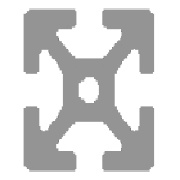
# Autodesk Inventor part: 40-4040
Saved by Autodesk Inventor 2016 (Build 200138000, 138)
## iProperties
IsCustomPart: 1
Created: 2015-07-26
Part Number: 40-4040
Material: Aluminum 6061
Document SubType Name: Modeling
Standard: 8020 Metric
Designer: myhome
Manufacturer: 8020
Standards Organization: 8020 Metric
Language: en-US
Size Designation: 40-4040
Categories: <MemberInstance><Categories><Category DisplayName="Structural Shapes" InternalName="089c4875-fa83-4c05-b084-43b9cc11f5ed" Mnemonic="GRDR"><CategoryParameter DisplayName="Mass per Length Unit" InternalName="0bb95a10-148f-4027-a459-38d7b056702a" Mnemonic="shpmass"/><CategoryParameter DisplayName="Section Area" InternalName="1ff91680-64b0-4202-b9a3-7fd3f94bba3b" Mnemonic="secarea"/><CategoryParameter DisplayName="Radius of Gyration (x)" InternalName="25778675-03e9-40c1-b6a8-4a9ed693320d" Mnemonic="gyrradx"/><CategoryParameter DisplayName="Torsional Rigidity Modulus" InternalName="26c1ec35-5026-4c63-ad0a-751cf684a536" Mnemonic="torrigmod"/><CategoryParameter DisplayName="Distance of the Center of Gravity X-X" InternalName="26c9bdb8-9c79-4b4f-a92e-8e197583c9c4" Mnemonic="grcendistX"/><CategoryParameter DisplayName="Legacy Member ID" InternalName="340afe4f-75d7-48d3-ab7d-943f3c3da468" Mnemonic="LegacyMemberID"/><CategoryParameter DisplayName="Base Length" InternalName="42e34263-8f20-4d0e-ad48-bf1385b87c24" Mnemonic="shplen"/><CategoryParameter DisplayName="Moment of Inertia (y)" InternalName="4b9f58ea-bced-460e-81ea-3d29ca5a49e3" Mnemonic="inermomy"/><CategoryParameter DisplayName="Moment of Inertia (x)" InternalName="4cd780bc-73d7-43ac-917a-579e5cbd684d" Mnemonic="inermomx"/><CategoryParameter DisplayName="Custom Base Point" InternalName="4f1d1b73-316d-484b-a3df-9cbabb16eb77" Mnemonic="shpBasePoint"/><CategoryParameter DisplayName="Shape Height" InternalName="50274e7d-5ac0-4796-92cb-c59e54983c67" Mnemonic="shpheig"/><CategoryParameter DisplayName="Section Module (y)" InternalName="59eaa5e9-d227-48dc-b6c1-6920f96e0f95" Mnemonic="secmody"/><CategoryParameter DisplayName="Section Designation" InternalName="5a64d034-428d-49c8-ba32-7619764de20f" Mnemonic="shpdes"/><CategoryParameter DisplayName="Section Module (x)" InternalName="72cfad18-cf51-4ed4-aaa7-c6b224f8419f" Mnemonic="secmodx"/><CategoryParameter DisplayName="Torsional Section Modulus" InternalName="7c55a8dc-8844-49f9-a867-cc677b30ec9a" Mnemonic="torsecmod"/><CategoryParameter DisplayName="Shape Width" InternalName="7c717d54-a18f-4666-b4d4-573cce22c62c" Mnemonic="shpwdth"/><CategoryParameter DisplayName="Second Shape Thickness" InternalName="9251a8e1-85fd-4e47-af99-afdb762317d9" Mnemonic="shpthick2"/><CategoryParameter DisplayName="FG Authored" InternalName="9c666724-f362-4ea7-ac62-f6a007de5c69" Mnemonic="shpFGAuto"/><CategoryParameter DisplayName="Distance of the Center of Gravity Y-Y" InternalName="bcc4fb17-7af4-436a-8f8c-d0aa3b0248c5" Mnemonic="grcendistY"/><CategoryParameter DisplayName="Radius of Gyration (y)" InternalName="bfa18ebe-1636-4dbe-8d42-b263e0b73184" Mnemonic="gyrrady"/><CategoryParameter DisplayName="Shape Thickness" InternalName="d109cf76-8eb4-42fc-9800-4409734adc67" Mnemonic="shpthick"/><CategoryParameter DisplayName="Coefficient of Shear Displacement" InternalName="de4c90c6-aaa8-468f-a335-6737b311b5d3" Mnemonic="shdispc"/><Category DisplayName="Other" InternalName="f02205ff-2390-476f-921c-0b3185f88e84" Mnemonic="OTHSHP"><CategoryParameter DisplayName="Moment of Inertia (y)" InternalName="044c654e-f649-48ac-84cc-650a29ae31ca" Mnemonic="inermomy"/><CategoryParameter DisplayName="Shape Thickness" InternalName="12b1a788-9233-48fd-a933-2df8ff42b15f" Mnemonic="shpthick"/><CategoryParameter DisplayName="Mass per Length Unit" InternalName="2fd289d6-9394-4d2d-97e6-6659d7d4551d" Mnemonic="shpmass"/><CategoryParameter DisplayName="Radius of Gyration (y)" InternalName="743e1dfe-1bba-408b-b985-cf752b207386" Mnemonic="gyrrady"/><CategoryParameter DisplayName="Section Module (y)" InternalName="88b8bff9-a616-4028-93d5-ed4f79680d13" Mnemonic="secmody"/><CategoryParameter DisplayName="Section Area" InternalName="c46ecdf8-b6eb-4db9-8b25-30258930c1e3" Mnemonic="secarea"/><CategoryParameter DisplayName="Section Module (x)" InternalName="cac70804-9d39-43bb-be17-56ea1f39a6c2" Mnemonic="secmodx"/><CategoryParameter DisplayName="Moment of Inertia (x)" InternalName="ec6737bc-264f-43ed-b0bd-f6d410c2718d" Mnemonic="inermomx"/><CategoryParameter DisplayName="Radius of Gyration (x)" InternalName="ee72c61e-565e-4fd6-b448-66e1e1abcb7e" Mnemonic="gyrradx"/><Category DisplayName="8020" InternalName="79851eee-1260-43d5-80eb-d25638456875" Mnemonic="8020"/></Category></Category><Category DisplayName="DataType" InternalName="23b78d0f-2648-40c6-8793-ca6db495c9e8" Mnemonic="DATATYPE"><CategoryParameter DisplayName="DisplayName" InternalName="05415f3d-3907-474b-a020-eb9d644f4cf3" Mnemonic="DISPLAYNAME"/><CategoryParameter DisplayName="Standard" InternalName="0c0a119c-1e12-4c84-803f-101930972f5e" Mnemonic="STANDARD"/><CategoryParameter DisplayName="Description" InternalName="13903e3d-64b1-4950-80da-f627842ea37f" Mnemonic="DESCRIPTION"/><CategoryParameter DisplayName="Designation" InternalName="2675968c-4ce5-49e0-a4f5-552d29089031" Mnemonic="DESIGNATION"/><CategoryParameter DisplayName="Default Row" InternalName="2af9ec52-faaa-4026-b378-f9fa4afca842" Mnemonic="DEFAULTROW"/><CategoryParameter DisplayName="Folder Name" InternalName="3f06958e-8713-4116-9be7-ed6184ecc97b" Mnemonic="FOLDERNAME"/><CategoryParameter DisplayName="Revision Guid" InternalName="45a75005-10b1-4dfc-8d6d-dfe629f0b93c" Mnemonic="REVISIONGUID"/><CategoryParameter DisplayName="FileName" InternalName="8b46a4cc-9585-4fed-90c3-899f57e09a73" Mnemonic="FILENAME"/><CategoryParameter DisplayName="StdsOrg" InternalName="8f5914e1-4693-403f-8ab5-d37768198c9d" Mnemonic="STDSORG"/><CategoryParameter DisplayName="Family Version" InternalName="914462f6-6e19-4b14-ba84-155b9680b1d0" Mnemonic="FAMILYREVISION"/><CategoryParameter DisplayName="Standard Revision" InternalName="91d5a463-65c2-4fde-b823-3b7fea5e8e17" Mnemonic="STANDARDREVISION"/><CategoryParameter DisplayName="Member Revision" InternalName="a65d44b9-392f-4f4f-857b-e4b3d54996fe" Mnemonic="MEMBERREVISION"/><CategoryParameter DisplayName="ClipFormat" InternalName="bc51e27b-3422-4e78-93ef-cec197ddf230" Mnemonic="CLIPFORMAT"/><CategoryParameter DisplayName="Manufacturer" InternalName="cd6c7a72-a28a-4e50-99a9-2c7f4e13e5ad" Mnemonic="MANUFACTURER"/><CategoryParameter DisplayName="InternalName" InternalName="cf1d0246-76d9-4b4a-8305-fa0409afb5c1" Mnemonic="INTERNALNAME"/><CategoryParameter DisplayName="IsMetric" InternalName="e2385c5b-1ea4-4823-96a8-8de651266ec3" Mnemonic="ISMETRIC"/><Category DisplayName="Part" InternalName="c0e0b642-3bcb-4cc8-9e80-f96d35c4afa4" Mnemonic="PART"><CategoryParameter DisplayName="Part Number" InternalName="016b6077-bfbe-49bd-92c9-d8d59c39c941" Mnemonic="PARTNUMBER"/><CategoryParameter DisplayName="Stock Number" InternalName="4dba7c1c-e26c-444e-836c-b08b433409a8" Mnemonic="STOCKNUMBER"/><CategoryParameter DisplayName="Material Key" InternalName="5c9a8adb-dd2b-4535-b97f-0a94a95fe41f" Mnemonic="MATERIALKEY"/><CategoryParameter DisplayName="Material" InternalName="818a152a-d3c3-49ca-80ee-df7d91421b8e" Mnemonic="MATERIAL"/></Category></Category></Categories><FamilyTemplate Id="40-4040"><FamilyTemplateParameters><FamilyTemplateParameter ObjectType="kModelParameterObject" ValueType="xs:double" Id="12" ObjectReferenceKey="Length"/><FamilyTemplateParameter ObjectType="kPartComponentDefinitionObject" ValueType="xs:string" Id="23" SubObjectId="Material"/><FamilyTemplateParameter ObjectType="kPropertyObject" ValueType="xs:string" Id="26" ObjectReferenceKey="{32853F0F-3444-11d1-9E93-0060B03C1CA6}" SubObjectId="5"/><FamilyTemplateParameter ObjectType="kPropertyObject" ValueType="xs:string" Id="27" ObjectReferenceKey="{32853F0F-3444-11d1-9E93-0060B03C1CA6}" SubObjectId="52"/></FamilyTemplateParameters></FamilyTemplate><CategoryParameterMap><ParamToTemplateMap><ParamToTemplate CategoryParameter="//CategoryParameter[@InternalName='cf1d0246-76d9-4b4a-8305-fa0409afb5c1']" ConstantValue="b86b142a-693f-4513-a498-88654243566b"/><ParamToTemplate CategoryParameter="//CategoryParameter[@InternalName='45a75005-10b1-4dfc-8d6d-dfe629f0b93c']" ConstantValue="d41eaa97-e16a-48df-8556-97121bae5127"/><ParamToTemplate CategoryParameter="//CategoryParameter[@InternalName='3f06958e-8713-4116-9be7-ed6184ecc97b']" ConstantValue="40-4040"/><ParamToTemplate CategoryParameter="//CategoryParameter[@InternalName='8f5914e1-4693-403f-8ab5-d37768198c9d']" ConstantValue="8020 Metric"/><ParamToTemplate CategoryParameter="//CategoryParameter[@InternalName='0c0a119c-1e12-4c84-803f-101930972f5e']" TemplateParameter="18"/><ParamToTemplate CategoryParameter="//CategoryParameter[@InternalName='91d5a463-65c2-4fde-b823-3b7fea5e8e17']" TemplateParameter="19"/><ParamToTemplate CategoryParameter="//CategoryParameter[@InternalName='cd6c7a72-a28a-4e50-99a9-2c7f4e13e5ad']" ConstantValue="8020"/><ParamToTemplate CategoryParameter="//CategoryParameter[@InternalName='13903e3d-64b1-4950-80da-f627842ea37f']" TemplateParameter="22"/><ParamToTemplate CategoryParameter="//CategoryParameter[@InternalName='05415f3d-3907-474b-a020-eb9d644f4cf3']" ConstantValue="40-4040"/><ParamToTemplate CategoryParameter="//CategoryParameter[@InternalName='914462f6-6e19-4b14-ba84-155b9680b1d0']" ConstantValue="11"/><ParamToTemplate CategoryParameter="//CategoryParameter[@InternalName='bc51e27b-3422-4e78-93ef-cec197ddf230']" ConstantValue="CF_INVENTOR.STDPARTS"/><ParamToTemplate CategoryParameter="//CategoryParameter[@InternalName='e2385c5b-1ea4-4823-96a8-8de651266ec3']" ConstantValue="false"/><ParamToTemplate CategoryParameter="//CategoryParameter[@InternalName='2af9ec52-faaa-4026-b378-f9fa4afca842']" ConstantValue="1"/><ParamToTemplate CategoryParameter="//CategoryParameter[@InternalName='9c666724-f362-4ea7-ac62-f6a007de5c69']" ConstantValue="1"/><ParamToTemplate CategoryParameter="//CategoryParameter[@InternalName='8b46a4cc-9585-4fed-90c3-899f57e09a73']" ConstantValue="40-4040"/><ParamToTemplate CategoryParameter="//CategoryParameter[@InternalName='a65d44b9-392f-4f4f-857b-e4b3d54996fe']" ConstantValue="2577b9ad-93dc-4f35-8dfb-0f20d1bb9b12"/><ParamToTemplate CategoryParameter="//CategoryParameter[@InternalName='a65d44b9-392f-4f4f-857b-e4b3d54996fe']" ConstantValue="2577b9ad-93dc-4f35-8dfb-0f20d1bb9b12"/><ParamToTemplate CategoryParameter="//CategoryParameter[@InternalName='2675968c-4ce5-49e0-a4f5-552d29089031']" TemplateParameter="27"/><ParamToTemplate CategoryParameter="//CategoryParameter[@InternalName='42e34263-8f20-4d0e-ad48-bf1385b87c24']" TemplateParameter="12"/><ParamToTemplate CategoryParameter="//CategoryParameter[@InternalName='818a152a-d3c3-49ca-80ee-df7d91421b8e']" TemplateParameter="23"/><ParamToTemplate CategoryParameter="//CategoryParameter[@InternalName='016b6077-bfbe-49bd-92c9-d8d59c39c941']" TemplateParameter="26"/></ParamToTemplateMap></CategoryParameterMap></MemberInstance>
Density: 2.7 g/cm^3
Appearance: Aluminum - Flat
Mass: 3601.23 g
Surface Area: 4954.89 cm^2
Volume: 1333.79 cm^3
_CCFamilyDisplayName: 40-4040
_FrameMemberDoc: Frame Member File
_Version: 15.0.0
_GetPNFromCC: 1
G_L: 59.055 in
G_W: 1.575 in
G_H: 1.575 in
Author: myhome
Autodesk Inventor part; units mm, degrees
ref_plane "YZ Plane" through (0, 0, 0) normal (1, 0, 0) x (0, 1, 0)
sketch "40-4040" plane through (0, 0, 0) normal (0, 0, 1) x (1, 0, 0)
  circle A0 centre (23.5106, 30.6383) radius 3.4
  line L0 (17.8806, 15.1137) -> (14.7956, 15.1137)
  arc A1 (13.2256, 16.6837) -> (14.7956, 15.1137) centre (14.7956, 16.6837) ccw
  line L1 (13.2256, 16.6837) -> (13.2256, 17.1458)
  arc A2 (13.4482, 17.6832) -> (13.2256, 17.1458) centre (13.9856, 17.1458) ccw
  line L2 (13.4482, 17.6832) -> (17.2935, 21.5285)
  arc A3 (20.7333, 22.9533) -> (17.2935, 21.5285) centre (20.7333, 18.0887) ccw
  line L3 (20.7333, 22.9533) -> (26.288, 22.9533)
  arc A4 (29.7277, 21.5285) -> (26.288, 22.9533) centre (26.288, 18.0887) ccw
  line L4 (29.7277, 21.5285) -> (33.573, 17.6832)
  arc A5 (33.7956, 17.1458) -> (33.573, 17.6832) centre (33.0356, 17.1458) ccw
  line L5 (33.7956, 17.1458) -> (33.7956, 16.6837)
  arc A6 (32.2256, 15.1137) -> (33.7956, 16.6837) centre (32.2256, 16.6837) ccw
  line L6 (32.2256, 15.1137) -> (29.1406, 15.1137)
  arc A7 (29.1406, 15.1137) -> (27.5706, 13.5437) centre (29.1406, 13.5437) ccw
  line L7 (27.5706, 13.5437) -> (27.5706, 12.2083)
  arc A8 (27.5706, 12.2083) -> (29.1406, 10.6383) centre (29.1406, 12.2083) ccw
  line L8 (29.1406, 10.6383) -> (40.3406, 10.6383)
  arc A9 (40.3406, 10.6383) -> (43.5106, 13.8083) centre (40.3406, 13.8083) ccw
  line L9 (43.5106, 13.8083) -> (43.5106, 25.0083)
  arc A10 (43.5106, 25.0083) -> (41.9406, 26.5783) centre (41.9406, 25.0083) ccw
  line L10 (41.9406, 26.5783) -> (40.7606, 26.5783)
  arc A11 (40.7606, 26.5783) -> (39.1906, 25.0083) centre (40.7606, 25.0083) ccw
  line L11 (39.1906, 25.0083) -> (39.1906, 21.9229)
  arc A12 (37.6206, 20.3529) -> (39.1906, 21.9229) centre (37.6206, 21.9229) ccw
  line L12 (37.6206, 20.3529) -> (37.1307, 20.3529)
  arc A13 (36.6743, 20.6913) -> (37.1307, 20.3529) centre (37.3223, 21.0883) ccw
  line L13 (36.6743, 20.6913) -> (32.5869, 24.7788)
  arc A14 (31.1956, 28.1375) -> (32.5869, 24.7788) centre (35.9456, 28.1375) ccw
  line L14 (31.1956, 28.1375) -> (31.1956, 33.1391)
  arc A15 (32.5869, 36.4978) -> (31.1956, 33.1391) centre (35.9456, 33.1391) ccw
  line L15 (32.5869, 36.4978) -> (36.7901, 40.7011)
  arc A16 (37.3275, 40.9237) -> (36.7901, 40.7011) centre (37.3275, 40.1637) ccw
  line L16 (37.3275, 40.9237) -> (37.6206, 40.9237)
  arc A17 (39.1906, 39.3537) -> (37.6206, 40.9237) centre (37.6206, 39.3537) ccw
  line L17 (39.1906, 39.3537) -> (39.1906, 36.2683)
  arc A18 (39.1906, 36.2683) -> (40.7606, 34.6983) centre (40.7606, 36.2683) ccw
  line L18 (40.7606, 34.6983) -> (41.9406, 34.6983)
  arc A19 (41.9406, 34.6983) -> (43.5106, 36.2683) centre (41.9406, 36.2683) ccw
  line L19 (43.5106, 36.2683) -> (43.5106, 47.4683)
  arc A20 (43.5106, 47.4683) -> (40.3406, 50.6383) centre (40.3406, 47.4683) ccw
  line L20 (40.3406, 50.6383) -> (29.1406, 50.6383)
  arc A21 (29.1406, 50.6383) -> (27.5706, 49.0683) centre (29.1406, 49.0683) ccw
  line L21 (27.5706, 49.0683) -> (27.5706, 47.7329)
  arc A22 (27.5706, 47.7329) -> (29.1406, 46.1629) centre (29.1406, 47.7329) ccw
  line L22 (29.1406, 46.1629) -> (32.2256, 46.1629)
  arc A23 (33.7956, 44.5929) -> (32.2256, 46.1629) centre (32.2256, 44.5929) ccw
  line L23 (33.7956, 44.5929) -> (33.7956, 44.1308)
  arc A24 (33.573, 43.5934) -> (33.7956, 44.1308) centre (33.0356, 44.1308) ccw
  line L24 (33.573, 43.5934) -> (29.7277, 39.7481)
  arc A25 (26.288, 38.3233) -> (29.7277, 39.7481) centre (26.288, 43.1878) ccw
  line L25 (26.288, 38.3233) -> (20.7333, 38.3233)
  arc A26 (17.2935, 39.7481) -> (20.7333, 38.3233) centre (20.7333, 43.1878) ccw
  line L26 (17.2935, 39.7481) -> (13.4482, 43.5934)
  arc A27 (13.2256, 44.1308) -> (13.4482, 43.5934) centre (13.9856, 44.1308) ccw
  line L27 (13.2256, 44.1308) -> (13.2256, 44.5929)
  arc A28 (14.7956, 46.1629) -> (13.2256, 44.5929) centre (14.7956, 44.5929) ccw
  line L28 (14.7956, 46.1629) -> (17.8806, 46.1629)
  arc A29 (17.8806, 46.1629) -> (19.4506, 47.7329) centre (17.8806, 47.7329) ccw
  line L29 (19.4506, 47.7329) -> (19.4506, 49.0683)
  arc A30 (19.4506, 49.0683) -> (17.8806, 50.6383) centre (17.8806, 49.0683) ccw
  line L30 (17.8806, 50.6383) -> (6.6806, 50.6383)
  arc A31 (6.6806, 50.6383) -> (3.5106, 47.4683) centre (6.6806, 47.4683) ccw
  line L31 (3.5106, 47.4683) -> (3.5106, 36.2113)
  arc A32 (3.5106, 36.2113) -> (5.0806, 34.6413) centre (5.0806, 36.2113) ccw
  line L32 (5.0806, 34.6413) -> (6.2606, 34.6413)
  arc A33 (6.2606, 34.6413) -> (7.8306, 36.2113) centre (6.2606, 36.2113) ccw
  line L33 (7.8306, 36.2113) -> (7.8306, 39.114)
  arc A34 (9.4554, 40.683) -> (7.8306, 39.114) centre (9.4006, 39.114) ccw
  line L34 (9.4554, 40.683) -> (9.7907, 40.6713)
  arc A35 (10.4701, 40.4621) -> (9.7907, 40.6713) centre (9.9327, 39.9247) ccw
  line L35 (10.4701, 40.4621) -> (14.4344, 36.4978)
  arc A36 (15.8256, 33.1391) -> (14.4344, 36.4978) centre (11.0756, 33.1391) ccw
  line L36 (15.8256, 33.1391) -> (15.8256, 28.1375)
  arc A37 (14.4344, 24.7788) -> (15.8256, 28.1375) centre (11.0756, 28.1375) ccw
  line L37 (14.4344, 24.7788) -> (10.2311, 20.5755)
  arc A38 (9.6937, 20.3529) -> (10.2311, 20.5755) centre (9.6937, 21.1129) ccw
  line L38 (9.6937, 20.3529) -> (9.4006, 20.3529)
  arc A39 (7.8306, 21.9229) -> (9.4006, 20.3529) centre (9.4006, 21.9229) ccw
  line L39 (7.8306, 21.9229) -> (7.8306, 24.8804)
  arc A40 (7.8306, 24.8804) -> (6.2606, 26.5178) centre (6.2621, 24.9478) ccw
  line L40 (6.2606, 26.5178) -> (5.0806, 26.5178)
  arc A41 (5.0806, 26.5178) -> (3.5106, 24.8804) centre (5.0792, 24.9478) ccw
  line L41 (3.5106, 24.8804) -> (3.5106, 13.6199)
  arc A42 (3.5106, 13.6199) -> (6.836, 10.6383) centre (6.6753, 13.8042) ccw
  line L42 (6.836, 10.6383) -> (17.8806, 10.6383)
  arc A43 (17.8806, 10.6383) -> (19.4506, 12.2083) centre (17.8806, 12.2083) ccw
  line L43 (19.4506, 12.2083) -> (19.4506, 13.5437)
  arc A44 (19.4506, 13.5437) -> (17.8806, 15.1137) centre (17.8806, 13.5437) ccw
  line L44 (23.5106, 30.6383) -> (23.5106, 33.1383)
  line L45 (23.5106, 30.6383) -> (21.0106, 30.6383)
  line L46 (23.5106, 30.6383) -> (23.5106, 28.1383)
  line L47 (23.5106, 30.6383) -> (26.0106, 30.6383)
  line L48 (23.5106, 35.6383) -> (23.5106, 36.5383)
  line L49 (18.5106, 30.6383) -> (17.6106, 30.6383)
  line L50 (23.5106, 25.6383) -> (23.5106, 24.7383)
  line L51 (28.5106, 30.6383) -> (29.4106, 30.6383)
ref_plane "Start Plane" through (0, 0, 0) normal (0, 0, 1) x (1, 0, 0)
ref_plane "End Plane" through (0, 0, 1500) normal (0, 0, 1) x (1, 0, 0)
sketch "Sketch" plane through (0, 0, 0) normal (0, 0, 1) x (1, 0, 0)
  circle A0 centre (0, 0) radius 3.4
  line L0 (-5.63, -15.5246) -> (-8.715, -15.5246)
  arc A1 (-10.285, -13.9546) -> (-8.715, -15.5246) centre (-8.715, -13.9546) ccw
  line L1 (-10.285, -13.9546) -> (-10.285, -13.4925)
  arc A2 (-10.0624, -12.9551) -> (-10.285, -13.4925) centre (-9.525, -13.4925) ccw
  line L2 (-10.0624, -12.9551) -> (-6.2171, -9.1098)
  arc A3 (-2.7773, -7.685) -> (-6.2171, -9.1098) centre (-2.7773, -12.5496) ccw
  line L3 (-2.7773, -7.685) -> (2.7773, -7.685)
  arc A4 (6.2171, -9.1098) -> (2.7773, -7.685) centre (2.7773, -12.5496) ccw
  line L4 (6.2171, -9.1098) -> (10.0624, -12.9551)
  arc A5 (10.285, -13.4925) -> (10.0624, -12.9551) centre (9.525, -13.4925) ccw
  line L5 (10.285, -13.4925) -> (10.285, -13.9546)
  arc A6 (8.715, -15.5246) -> (10.285, -13.9546) centre (8.715, -13.9546) ccw
  line L6 (8.715, -15.5246) -> (5.63, -15.5246)
  arc A7 (5.63, -15.5246) -> (4.06, -17.0946) centre (5.63, -17.0946) ccw
  line L7 (4.06, -17.0946) -> (4.06, -18.43)
  arc A8 (4.06, -18.43) -> (5.63, -20) centre (5.63, -18.43) ccw
  line L8 (5.63, -20) -> (16.83, -20)
  arc A9 (16.83, -20) -> (20, -16.83) centre (16.83, -16.83) ccw
  line L9 (20, -16.83) -> (20, -5.63)
  arc A10 (20, -5.63) -> (18.43, -4.06) centre (18.43, -5.63) ccw
  line L10 (18.43, -4.06) -> (17.25, -4.06)
  arc A11 (17.25, -4.06) -> (15.68, -5.63) centre (17.25, -5.63) ccw
  line L11 (15.68, -5.63) -> (15.68, -8.7154)
  arc A12 (14.11, -10.2854) -> (15.68, -8.7154) centre (14.11, -8.7154) ccw
  line L12 (14.11, -10.2854) -> (13.6201, -10.2854)
  arc A13 (13.1637, -9.947) -> (13.6201, -10.2854) centre (13.8117, -9.55) ccw
  line L13 (13.1637, -9.947) -> (9.0762, -5.8595)
  arc A14 (7.685, -2.5008) -> (9.0762, -5.8595) centre (12.435, -2.5008) ccw
  line L14 (7.685, -2.5008) -> (7.685, 2.5008)
  arc A15 (9.0762, 5.8595) -> (7.685, 2.5008) centre (12.435, 2.5008) ccw
  line L15 (9.0762, 5.8595) -> (13.2795, 10.0628)
  arc A16 (13.8169, 10.2854) -> (13.2795, 10.0628) centre (13.8169, 9.5254) ccw
  line L16 (13.8169, 10.2854) -> (14.11, 10.2854)
  arc A17 (15.68, 8.7154) -> (14.11, 10.2854) centre (14.11, 8.7154) ccw
  line L17 (15.68, 8.7154) -> (15.68, 5.63)
  arc A18 (15.68, 5.63) -> (17.25, 4.06) centre (17.25, 5.63) ccw
  line L18 (17.25, 4.06) -> (18.43, 4.06)
  arc A19 (18.43, 4.06) -> (20, 5.63) centre (18.43, 5.63) ccw
  line L19 (20, 5.63) -> (20, 16.83)
  arc A20 (20, 16.83) -> (16.83, 20) centre (16.83, 16.83) ccw
  line L20 (16.83, 20) -> (5.63, 20)
  arc A21 (5.63, 20) -> (4.06, 18.43) centre (5.63, 18.43) ccw
  line L21 (4.06, 18.43) -> (4.06, 17.0946)
  arc A22 (4.06, 17.0946) -> (5.63, 15.5246) centre (5.63, 17.0946) ccw
  line L22 (5.63, 15.5246) -> (8.715, 15.5246)
  arc A23 (10.285, 13.9546) -> (8.715, 15.5246) centre (8.715, 13.9546) ccw
  line L23 (10.285, 13.9546) -> (10.285, 13.4925)
  arc A24 (10.0624, 12.9551) -> (10.285, 13.4925) centre (9.525, 13.4925) ccw
  line L24 (10.0624, 12.9551) -> (6.2171, 9.1098)
  arc A25 (2.7773, 7.685) -> (6.2171, 9.1098) centre (2.7773, 12.5496) ccw
  line L25 (2.7773, 7.685) -> (-2.7773, 7.685)
  arc A26 (-6.2171, 9.1098) -> (-2.7773, 7.685) centre (-2.7773, 12.5496) ccw
  line L26 (-6.2171, 9.1098) -> (-10.0624, 12.9551)
  arc A27 (-10.285, 13.4925) -> (-10.0624, 12.9551) centre (-9.525, 13.4925) ccw
  line L27 (-10.285, 13.4925) -> (-10.285, 13.9546)
  arc A28 (-8.715, 15.5246) -> (-10.285, 13.9546) centre (-8.715, 13.9546) ccw
  line L28 (-8.715, 15.5246) -> (-5.63, 15.5246)
  arc A29 (-5.63, 15.5246) -> (-4.06, 17.0946) centre (-5.63, 17.0946) ccw
  line L29 (-4.06, 17.0946) -> (-4.06, 18.43)
  arc A30 (-4.06, 18.43) -> (-5.63, 20) centre (-5.63, 18.43) ccw
  line L30 (-5.63, 20) -> (-16.83, 20)
  arc A31 (-16.83, 20) -> (-20, 16.83) centre (-16.83, 16.83) ccw
  line L31 (-20, 16.83) -> (-20, 5.573)
  arc A32 (-20, 5.573) -> (-18.43, 4.003) centre (-18.43, 5.573) ccw
  line L32 (-18.43, 4.003) -> (-17.25, 4.003)
  arc A33 (-17.25, 4.003) -> (-15.68, 5.573) centre (-17.25, 5.573) ccw
  line L33 (-15.68, 5.573) -> (-15.68, 8.4757)
  arc A34 (-14.0552, 10.0447) -> (-15.68, 8.4757) centre (-14.11, 8.4757) ccw
  line L34 (-14.0552, 10.0447) -> (-13.7199, 10.033)
  arc A35 (-13.0405, 9.8238) -> (-13.7199, 10.033) centre (-13.5779, 9.2864) ccw
  line L35 (-13.0405, 9.8238) -> (-9.0762, 5.8595)
  arc A36 (-7.685, 2.5008) -> (-9.0762, 5.8595) centre (-12.435, 2.5008) ccw
  line L36 (-7.685, 2.5008) -> (-7.685, -2.5008)
  arc A37 (-9.0762, -5.8595) -> (-7.685, -2.5008) centre (-12.435, -2.5008) ccw
  line L37 (-9.0762, -5.8595) -> (-13.2795, -10.0628)
  arc A38 (-13.8169, -10.2854) -> (-13.2795, -10.0628) centre (-13.8169, -9.5254) ccw
  line L38 (-13.8169, -10.2854) -> (-14.11, -10.2854)
  arc A39 (-15.68, -8.7154) -> (-14.11, -10.2854) centre (-14.11, -8.7154) ccw
  line L39 (-15.68, -8.7154) -> (-15.68, -5.7579)
  arc A40 (-15.68, -5.7579) -> (-17.25, -4.1204) centre (-17.2485, -5.6904) ccw
  line L40 (-17.25, -4.1204) -> (-18.43, -4.1204)
  arc A41 (-18.43, -4.1204) -> (-20, -5.7579) centre (-18.4315, -5.6904) ccw
  line L41 (-20, -5.7579) -> (-20, -17.0184)
  arc A42 (-20, -17.0184) -> (-16.6746, -20) centre (-16.8354, -16.8341) ccw
  line L42 (-16.6746, -20) -> (-5.63, -20)
  arc A43 (-5.63, -20) -> (-4.06, -18.43) centre (-5.63, -18.43) ccw
  line L43 (-4.06, -18.43) -> (-4.06, -17.0946)
  arc A44 (-4.06, -17.0946) -> (-5.63, -15.5246) centre (-5.63, -17.0946) ccw
  line L44 (0, 0) -> (0, 2.5)
  line L45 (0, 0) -> (-2.5, 0)
  line L46 (0, 0) -> (0, -2.5)
  line L47 (0, 0) -> (2.5, 0)
  line L48 (0, 5) -> (0, 5.9)
  line L49 (-5, 0) -> (-5.9, 0)
  line L50 (0, -5) -> (0, -5.9)
  line L51 (5, 0) -> (5.9, 0)
  constraints: 1 other
extrude "Body" add sketch "Sketch" along normal up to surface (1500 mm away) from surface at 0
sketch "Sketch2" plane through (0, 0, 0) normal (0, 0, 1) x (1, 0, 0)
  line L0 (0, 0) -> (10, 0)
ref_plane "Work Plane3" through (0, 0, 0) normal (0, -1, 0) x (1, 0, 0)
sketch "Sketch3" plane through (0, 0, 0) normal (0, -1, 0) x (1, 0, 0)
  line L0 (-2, 0) -> (12, 0)
  line L1 (-2, 1500) -> (12, 1500)
  dimension "d7" = 1500
  measures "d7" distance between parallel lines of L0 L1
equation "\"G_OFFSET_START\" = 0"
equation "\"G_OFFSET_END\" = 0"
equation "\"G_L\" = d7"
body "Solid1"
